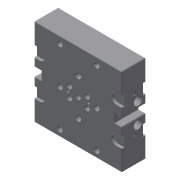
# Autodesk Inventor part: topplate2
Saved by Autodesk Inventor 2022 (Build 260148000, 148)
## iProperties
Shininess: 64.0
Length Units: 11269
Angle Units: 11279
Time Units: 11290
Mass Units: 11283
Length Display Precision: 3
Angle Display Precision: 2
Compacted: True
Part Number: topplate2
Document SubType Name: Modeling
Created: 2003-04-03
Designer: Sudhir John
Density: 1 g/cm^3
Material: Generic
Appearance: Default
Density: 0.0
Volumn: 0.0
Area: 0.0
PropertySet Name: Model Information
Control State: 0
Master: False
Checked Out: False
Author: Sudhir John
Autodesk Inventor part; units mm, degrees
sketch "Sketch1" plane through (0, 0, 0) normal (0, 0, 1) x (1, 0, 0)
  line L0 (-26.8734, 25.9044) -> (176.3266, 25.9044)
  line L1 (176.3266, 25.9044) -> (176.3266, -177.2956)
  line L2 (176.3266, -177.2956) -> (-26.8734, -177.2956)
  line L3 (-26.8734, -177.2956) -> (-26.8734, 25.9044)
  dimension "d0" = 203.2
  dimension "d1" = 203.2
  constraints: 8 end point, 2 parallel, 1 horizontal, 1 perpendicular
  measures "d0" distance of L0.start L0.end
  measures "d1" distance of L2.end L0.start
extrude "Extrusion1" add sketch "Sketch1" along normal blind 55.4482
ref_plane "Work Plane1" through (74.7266, -177.2956, 0) normal (1, 0, 0) x (0, 0, -1)
ref_plane "Work Plane2" through (-26.8734, -75.6956, 55.4482) normal (0, 1, 0) x (1, 0, 0)
sketch "Sketch3" plane through (0, 0, 55.4482) normal (0, 0, 1) x (1, 0, 0)
  line L0 (-26.8734, -177.2956) -> (-26.8734, 25.9044) projected
  line L1 (-47.1934, -75.6956) -> (237.2866, -75.6956) projected
  line L2 (-26.8734, -66.1706) -> (-10.8714, -66.1706)
  line L3 (-10.8714, -66.1706) -> (-10.8714, -85.2206)
  line L4 (-10.8714, -85.2206) -> (-26.8734, -85.2206)
  line L5 (-26.8734, -85.2206) -> (-26.8734, -66.1706)
  dimension "d9" = 19.05
  dimension "d10" = 9.525
  dimension "d11" = 16.002
  constraints: 8 end point, 2 parallel, 1 horizontal, 1 perpendicular, 1 point on line
  measures "d9" distance of L2.end L3.end
  measures "d10" distance between parallel lines of L2 L1
  measures "d11" distance of L3.end L4.end
extrude "Extrusion3" cut sketch "Sketch3" against normal through all
mirror "Mirror2" about plane through (74.7266, -177.2956, 0) normal (1, 0, 0) of "Extrusion3"
sketch "Sketch6" plane through (0, 0, 55.4482) normal (0, 0, 1) x (1, 0, 0)
  line L0 (-26.8734, -177.2956) -> (-26.8734, -85.2206) projected
  line L1 (49.3266, -177.2956) -> (-26.8734, -177.2956) projected
  line L2 (-26.8734, -129.6706) -> (-14.1734, -129.6706)
  line L3 (-14.1734, -104.2706) -> (-26.8734, -104.2706)
  arc A0 (-14.1734, -129.6706) -> (-14.1734, -104.2706) centre (-14.1734, -116.9706) ccw
  dimension "d30" = 47.625
  dimension "d32" = 12.7
  dimension "d33" = 25.4
  constraints: 4 end point, 2 point on circle, 2 point on line, 2 tangent, 1 centre point, 1 parallel
  measures "d30" distance between parallel lines of L1 L2
  measures "d32" distance of L3.start L3.end
  measures "d33" distance of L3.end L2.start
extrude "Extrusion4" cut sketch "Sketch6" against normal blind 6.35
mirror "Mirror3" about plane through (74.7266, -177.2956, 0) normal (1, 0, 0) of "Extrusion4"
mirror "Mirror4" about plane through (-26.8734, -75.6956, 55.4482) normal (0, 1, 0) of "Extrusion4", "Mirror3"
sketch "Sketch7" plane through (0, 0, 0) normal (0, 0, -1) x (-1, 0, 0)
  line L0 (-176.3266, -85.2206) -> (-176.3266, -177.2956) projected
  line L1 (-176.3266, -177.2956) -> (-100.1266, -177.2956) projected
  line L2 (-74.7266, -197.6156) -> (-74.7266, 86.8644) projected
  line L3 (-237.2866, -75.6956) -> (47.1934, -75.6956) projected
  point P0 (-117.5891, -161.4206)
  point P1 (-31.8641, -161.4206)
  point P2 (-117.5891, 10.0294)
  point P3 (-31.8641, 10.0294)
  point P4 (-117.5891, -75.6956)
  point P5 (-31.8641, -75.6956)
  point P6 (-74.7266, -118.5581)
  point P7 (-74.7266, -32.8331)
  dimension "d36" = 15.875
  dimension "d37" = 58.7375
  constraints: 4 point on line, 3 symmetric about line
  measures "d36" distance from line of L1 point (-117.589, -161.421)
  measures "d37" distance from line of L0 point (-117.589, -161.421)
hole "Hole3" at (117.5891, -161.4206, 0) at (31.8641, -161.4206, 0) at (117.5891, 10.0294, 0) at (31.8641, 10.0294, 0) at (117.5891, -75.6956, 0) at (31.8641, -75.6956, 0) at (74.7266, -118.5581, 0) at (74.7266, -32.8331, 0) direction (0, 0, 1) diameter 13.4874 end through all counterbore diameter 19.8374 counterbore depth 14.224
sketch "Sketch8" plane through (0, 0, 55.4482) normal (0, 0, 1) x (1, 0, 0)
  point P0 (74.7266, -75.6956)
hole "Hole4" at (74.7266, -75.6956, 55.4482) direction (0, 0, -1) diameter 11.938 end through all
sketch "Sketch9" plane through (0, 0, 55.4482) normal (0, 0, 1) x (1, 0, 0)
  circle A0 centre (74.7266, -75.6956) radius 5.969 projected
  line L0 (74.7266, 86.8644) -> (74.7266, -197.6156) projected
  line L1 (-47.1934, -75.6956) -> (237.2866, -75.6956) projected
  point P0 (54.1526, -87.6336)
  point P1 (95.3006, -87.6336)
  point P2 (54.1526, -63.7576)
  point P3 (95.3006, -63.7576)
  dimension "d52" = 20.574
  dimension "d53" = 11.938
  constraints: 3 symmetric about line
  measures "d52" horizontal distance of A0.centre point (54.153, -87.634)
  measures "d53" vertical distance of A0.centre point (54.153, -87.634)
hole "Hole5" at (54.1526, -87.6336, 55.4482) at (95.3006, -87.6336, 55.4482) at (54.1526, -63.7576, 55.4482) at (95.3006, -63.7576, 55.4482) direction (0, 0, -1) diameter 8.7122 end through all counterbore diameter 12.7 counterbore depth 8.7122
sketch "Sketch10" plane through (0, 0, 0) normal (0, 0, -1) x (-1, 0, 0)
  circle A0 centre (-74.7266, -75.6956) radius 5.969 projected
  line L0 (-74.7266, -197.6156) -> (-74.7266, 86.8644) projected
  point P0 (-98.5264, -75.6956)
  point P1 (-50.9268, -75.6956)
  dimension "d61" = 23.7998
  constraints: 1 symmetric about line
  measures "d61" distance of A0.centre point (-98.526, -75.696)
hole "Hole6" at (98.5264, -75.6956, 0) at (50.9268, -75.6956, 0) direction (0, 0, 1) diameter 6.35 end through all counterbore diameter 7.9375 counterbore depth 13.462
sketch "Sketch11" plane through (176.3266, 25.9044, 55.4482) normal (1, 0, 0) x (0, 0, -1)
  line L0 (55.4482, 0) -> (55.4482, -92.075) projected
  line L1 (-16.6345, -101.6) -> (60.993, -101.6) projected
  point P0 (37.2872, -77.978)
  point P1 (37.2872, -125.222)
  dimension "d69" = 23.622
  dimension "d70" = 18.161
  constraints: 1 symmetric about line
  measures "d69" distance from line of L1 point (37.287, -77.978)
  measures "d70" distance from line of L0 point (37.287, -77.978)
hole "Hole7" at (176.3266, -52.0736, 18.161) at (176.3266, -99.3176, 18.161) direction (-1, 0, 0) diameter 8.6868 depth 104.775 tip angle 118 counterbore diameter 19.05 counterbore depth 17.4625
sketch "Sketch12" plane through (176.3266, 25.9044, 55.4482) normal (1, 0, 0) x (0, 0, -1)
  line L0 (55.4482, 0) -> (55.4482, -92.075) projected
  line L1 (-16.6345, -101.6) -> (60.993, -101.6) projected
  point P0 (30.0482, -60.325)
  point P1 (30.0482, -142.875)
  dimension "d78" = 41.275
  dimension "d79" = 25.4
  constraints: 1 symmetric about line
  measures "d78" distance from line of L1 point (30.048, -60.325)
  measures "d79" distance from line of L0 point (30.048, -60.325)
hole "Hole8" at (176.3266, -34.4206, 25.4) at (176.3266, -116.9706, 25.4) direction (-1, 0, 0) diameter 7.7978 depth 32.4612 tip angle 118 thread size "3/8-16 UNC" class "1B" standard "ANSI Unified Screw Threads"
mirror "Mirror5" about plane through (74.7266, -177.2956, 0) normal (1, 0, 0) of "Hole8"
sketch "Sketch13" plane through (160.3246, -85.2206, 0) normal (1, 0, 0) x (0, 0, -1)
  line L0 (-55.4482, 0) -> (-55.4482, 19.05) projected
  line L1 (-72.0827, 9.525) -> (5.5448, 9.525) projected
  point P0 (-42.7482, 9.525)
  point P1 (-17.3482, 9.525)
  dimension "d87" = 12.7
  dimension "d88" = 25.4
  constraints: 2 point on line
  measures "d87" distance from line of point (-42.748, 9.525) L0
  measures "d88" distance of point (-17.348, 9.525) point (-42.748, 9.525)
hole "Hole9" at (160.3246, -75.6956, 42.7482) at (160.3246, -75.6956, 17.3482) direction (-1, 0, 0) diameter 7.7978 depth 15.24 tip angle 118 thread size "3/8-16 UNC" class "1B" standard "ANSI Unified Screw Threads"
mirror "Mirror6" about plane through (74.7266, -177.2956, 0) normal (1, 0, 0) of "Hole9"
ref_plane "Work Plane3" through (0, 0, 27.7241) normal (0, 0, 1) x (1, 0, 0)
mirror "Mirror7" about plane through (0, 0, 27.7241) normal (0, 0, 1) of "Extrusion4", "Mirror3", "Mirror4"
chamfer "Chamfer1" distance 1.27 angle 45 39 edges at (74.7266, 25.9044, 55.4482) (176.3266, 25.9044, 27.7241) (74.7266, 25.9044, 0) (-26.8734, 25.9044, 27.7241) (-26.8734, 2.0919, 55.4482) (-26.8734, -56.6456, 55.4482) (-26.8734, -94.7456, 55.4482) (-26.8734, -153.4831, 55.4482) (74.7266, -177.2956, 55.4482) (176.3266, -153.4831, 55.4482) (176.3266, -94.7456, 55.4482) (176.3266, -56.6456, 55.4482) (176.3266, 2.0919, 55.4482) (176.3266, -177.2956, 27.7241) (176.3266, -153.4831, 0) (176.3266, -94.7456, 0) (176.3266, -56.6456, 0) (176.3266, 2.0919, 0) (-26.8734, 2.0919, 0) (-26.8734, -56.6456, 0) (-26.8734, -94.7456, 0) (-26.8734, -153.4831, 0) (74.7266, -177.2956, 0) (176.3266, -85.2206, 27.7241) (176.3266, -66.1706, 27.7241) (168.3256, -66.1706, 55.4482) (160.3246, -75.6956, 55.4482) (168.3256, -85.2206, 55.4482) (-10.8714, -75.6956, 55.4482) (-18.8724, -85.2206, 55.4482) (-18.8724, -66.1706, 55.4482) (-26.8734, -85.2206, 27.7241) (-26.8734, -66.1706, 27.7241) (-18.8724, -66.1706, 0) (-10.8714, -75.6956, 0) (-18.8724, -85.2206, 0) (168.3256, -85.2206, 0) (160.3246, -75.6956, 0) (168.3256, -66.1706, 0)
equation "\"d10\" = 0.5 * d9"
body "Solid1"
